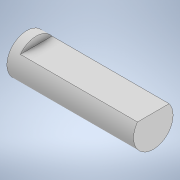
# Autodesk Inventor part: GA12-N20微型减速直流电机转动轴
Saved by Autodesk Inventor 2022 (Build 260153000, 153)
## iProperties
Created: 2022-05-21
Part Number: GA12-N20微型减速直流电机转动轴
Material: 常规
Document SubType Name: Modeling
Designer: zhcne
Density: 1 g/cm^3
Appearance: 默认
Author: zhcne
Autodesk Inventor part; units mm, degrees
ref_plane "YZ Plane" through (0, 0, 0) normal (1, 0, 0) x (0, 1, 0)
ref_plane "XZ Plane" through (0, 0, 0) normal (0, 1, 0) x (-1, 0, 0)
ref_plane "XY Plane" through (0, 0, 0) normal (0, 0, 1) x (1, 0, 0)
sketch "草图1" plane through (0, 0, 0) normal (1, 0, 0) x (0, 1, 0)
  circle A0 centre (0, 0) radius 1.25
  dimension "d0" = 2.5
  constraints: 1 centre point, 1 coincident
  measures "d0" diameter of A0
extrude "拉伸1" add sketch "草图1" along normal blind 0.6
sketch "草图2" plane through (0.6, 0, 0) normal (1, 0, 0) x (0, 0, -1)
  arc A0 (-1, 0.75) -> (1, 0.75) centre (0, 0) ccw
  circle A1 centre (0, 0) radius 1.25 projected
  line L0 (-1, 0.75) -> (1, 0.75)
  dimension "d3" = 2
  constraints: 4 point on circle, 2 end point, 1 centre point, 1 coincident, 1 horizontal
extrude "拉伸2" add sketch "草图2" along normal blind 7.4 contours L0 A0
